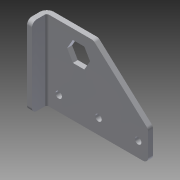
# Autodesk Inventor part: Spacer 3 (R-R) ipt
Saved by Autodesk Inventor 2014 (Build 180170000, 170)
## iProperties
Created: 2014-01-17
Part Number: Spacer 3 (R-R) ipt
Material: Aluminum 6061
Document SubType Name: Sheet Metal
Designer: Michael
Density: 2.71 g/cm^3
Sheet Metal Rule: Default
Appearance: Aluminum - Flat
Mass: 33.4634 g
Surface Area: 88.4494 cm^2
Volume: 12.3481 cm^3
Author: Michael
Autodesk Inventor part; units mm, degrees
ref_plane "YZ Plane" through (0, 0, 0) normal (1, 0, 0) x (0, 1, 0)
ref_plane "XZ Plane" through (0, 0, 0) normal (0, 1, 0) x (-1, 0, 0)
ref_plane "XY Plane" through (0, 0, 0) normal (0, 0, 1) x (1, 0, 0)
sketch "Sketch1" plane through (0, 0, 0) normal (0, 0, 1) x (1, 0, 0)
  line L0 (0, 0) -> (63.5, 0)
  line L1 (63.5, 0) -> (63.5, 19.05)
  line L2 (0, 50.8) -> (0, 0)
  circle A0 centre (6.35, 9.525) radius 2.0701
  circle A1 centre (31.75, 9.525) radius 2.0701
  circle A2 centre (57.15, 9.525) radius 2.0701
  line L3 (63.5, 19.05) -> (28.575, 50.8)
  line L4 (28.575, 50.8) -> (0, 50.8)
  line L5 (22.7162, 44.45) -> (26.3823, 38.1)
  line L6 (26.3823, 38.1) -> (22.7162, 31.75)
  line L7 (22.7162, 31.75) -> (15.3838, 31.75)
  line L8 (15.3838, 31.75) -> (11.7177, 38.1)
  line L9 (11.7177, 38.1) -> (15.3838, 44.45)
  line L10 (15.3838, 44.45) -> (22.7162, 44.45)
  point P0 (19.05, 38.1)
  dimension "d5" = 63.5
  dimension "d6" = 4.1402
  dimension "d7" = 6.35
  dimension "d8" = 9.525
  dimension "d24" = 25.4
  dimension "d29" = 50.8
  dimension "d30" = 19.05
  dimension "d31" = 28.575
  dimension "d32" = 12.7
  dimension "d34" = 19.05
  dimension "d35" = 12.7
  measures "d5" distance of L0.start L0.end
  measures "d6" diameter of A0
  measures "d7" distance from line of L2 A0.centre
  measures "d8" distance from line of L0 A0.centre
  measures "d24" distance of A0.centre A1.centre
  measures "d29" distance of L2.start L0.start
  measures "d30" distance of L0.end L1.end
  measures "d31" distance of L3.end L2.start
  measures "d32" distance between parallel lines of L7 L10
  measures "d34" distance from line of L2 point (19.05, 38.1)
  measures "d35" distance from line of L4 point (19.05, 38.1)
extrude "Plate1" add sketch "Sketch1" along normal blind 3.175
sketch "Sketch3" plane through (-1.27, 0, 4.445) normal (-1, 0, 0) x (0, -1, 0)
  line L0 (-50.8, 0) -> (0, 0)
  line L1 (0, 0) -> (0, 8.255)
  line L2 (0, 8.255) -> (-50.8, 8.255)
  line L3 (-50.8, 8.255) -> (-50.8, 0)
  constraints: 6 end point, 1 horizontal, 1 perpendicular, 1 vertical
edge flange "Flange2" height 12.7 angle 90 thickness 3.175 bend radius 1.27 thickness toward (-1, 0, 0) relief straight relief width 3.175 relief depth 1.5875 edges at (0, 25.4, 3.175) wall of the first edge with corners at (-1.27, 50.8, 4.445) (-1.27, 0, 4.445) (-1.27, 0, 12.7) (-1.27, 50.8, 12.7)
bend "Bend2"
corner "Corner2"
fillet "Fillet1" radius 3.175 5 edges at (28.575, 50.8, 1.5875) (-2.8575, 50.8, 12.7) (63.5, 19.05, 1.5875) (63.5, 0, 1.5875) (-2.8575, 0, 12.7)
equation "\"d36\" = BendReliefWidth"
equation "\"d37\" = BendReliefDepth"
equation "\"d38\" = MinimumRemnant"
equation "\"d39\" = BendRadius"
equation "\"d43\" = CornerReliefSize"
equation "\"d44\" = GapSize"
equation "\"d45\" = JacobiRadiusSize"
equation "\"BendRadius\" = Thickness"
equation "\"BendReliefWidth\" = Thickness"
equation "\"BendReliefDepth\" = 0.5 * Thickness"
equation "\"CornerReliefSize\" = 4 * Thickness"
equation "\"MinimumRemnant\" = 2 * Thickness"
equation "\"TransitionRadius\" = BendRadius"
equation "\"JacobiRadiusSize\" = BendRadius"
equation "\"GapSize\" = Thickness"
equation "\"d11\" = BendRadius"
equation "\"Thickness\" = 3.175"
body "Solid1"
